joystick (Autodesk Fusion 360 design; units mm, degrees)
Autodesk Fusion 360 part; units mm, degrees
sketch "Sketch1" plane through (0, 0, 0) normal (0, 1, 0) x (1, 0, 0)
  line L0 (0, 0) -> (-17.5, 0)
  line L1 (-17.5, 0) -> (-17.5, -17.5)
  line L2 (-17.5, -17.5) -> (0, -17.5)
  line L3 (0, -17.5) -> (0, 0)
  dimension "d1" = 17.5
  dimension "d2" = 17.5
  constraint horizontal L0
  constraint vertical L1
  constraint horizontal L2
  constraint vertical L3
  constraint coincident L0.start L3.end
  measures "d1" distance of L0.start L2.end
  measures "d2" distance of L1.end L2.end
extrude "Extrude1" add sketch "Sketch1" along normal blind 11
sketch "Sketch2" plane through (0, 11, 0) normal (0, 1, 0) x (-1, 0, 0)
  line L0 (0, 17.5) -> (0, 0)
  line L1 (0, 0) -> (17.5, 0)
  line L2 (17.5, 0) -> (17.5, 17.5)
  line L3 (17.5, 17.5) -> (0, 17.5)
  line L4 (7.85, 9.3) -> (9.65, 9.3)
  line L5 (9.65, 9.3) -> (9.65, 8.2)
  line L6 (9.65, 8.2) -> (7.85, 8.2)
  line L7 (7.85, 8.2) -> (7.85, 9.3)
  line L8 (8.75, 9.3) -> (8.75, 8.2)
  line L9 (9.65, 8.75) -> (7.85, 8.75)
  line L10 (0, 17.5) -> (17.5, 17.5)
  line L11 (0, 17.5) -> (0, 0)
  line L12 (8.75, 17.5) -> (8.75, 0)
  line L13 (0, 8.75) -> (17.5, 8.75)
  dimension "d5" = 1.8
  dimension "d6" = 1.1
  constraint horizontal L4
  constraint vertical L5
  constraint horizontal L6
  constraint vertical L7
  constraint midpoint L4 L8.start
  constraint midpoint L6 L8.end
  constraint midpoint L5 L9.start
  constraint midpoint L7 L9.end
  constraint coincident L0.start L3.end
  constraint coincident L2.end L3.start
  constraint coincident L0.end L1.start
  constraint midpoint L10 L12.start
  constraint midpoint L1 L12.end
  constraint midpoint L0 L13.start
  constraint midpoint L2 L13.end
  constraint collinear L9 L13
  constraint collinear L8 L12
  measures "d5" distance of L4.start L4.end
  measures "d6" distance of L4.end L5.end
extrude "Extrude2" add sketch "Sketch2" along normal blind 8 contours L6 L7 L8 L9 L12 L13 | L4 L7 L8 L9 L12 L13 | L4 L5 L8 L9 L12 L13 | L5 L6 L8 L9 L12 L13
sketch "Sketch3" plane through (0, 0, 0) normal (1, 0, 0) x (0, 1, 0)
  line L0 (0, 17.5) -> (0, 0)
  line L1 (0, 0) -> (11, 0)
  line L2 (11, 0) -> (11, 17.5)
  line L3 (11, 17.5) -> (0, 17.5)
  line L4 (0, 13.75) -> (11, 13.75)
  line L5 (11, 13.75) -> (11, 3.75)
  line L6 (11, 3.75) -> (0, 3.75)
  line L7 (0, 3.75) -> (0, 13.75)
  line L8 (11, 8.75) -> (0, 8.75)
  line L9 (11, 17.5) -> (11, 0)
  line L10 (11, 8.75) -> (0, 8.75)
  dimension "d11" = 10
  dimension "d12" = 11
  constraint horizontal L4
  constraint vertical L5
  constraint horizontal L6
  constraint vertical L7
  constraint coincident L0 L4.start
  constraint midpoint L5 L8.start
  constraint midpoint L7 L8.end
  constraint coincident L2.end L3.start
  constraint coincident L1.end L2.start
  constraint midpoint L9 L8.start
  constraint midpoint L0 L8.end
  constraint collinear L8 L10
  measures "d11" distance of L4 L6
  measures "d12" distance of L5.end L6.end
extrude "Extrude3" add sketch "Sketch3" along normal blind 3.5 contours L0 L2 L4 L5 L7 L8 L9 L10 | L0 L2 L5 L6 L7 L8 L9 L10
sketch "Sketch4" plane through (0, 0, 17.5) normal (0, 0, 1) x (-1, 0, 0)
  line L0 (17.5, 0) -> (0, 0)
  line L1 (0, 0) -> (0, -11)
  line L2 (0, -11) -> (17.5, -11)
  line L3 (17.5, -11) -> (17.5, 0)
  line L4 (14.25, -11) -> (3.25, -11)
  line L5 (3.25, -11) -> (3.25, 0)
  line L6 (3.25, 0) -> (14.25, 0)
  line L7 (14.25, 0) -> (14.25, -11)
  line L8 (8.75, -11) -> (8.75, 0)
  line L9 (17.5, -11) -> (0, -11)
  line L10 (8.75, -11) -> (8.75, 0)
  dimension "d18" = 11
  constraint horizontal L4
  constraint vertical L5
  constraint horizontal L6
  constraint vertical L7
  constraint coincident L0 L5.end
  constraint coincident L2 L4.start
  constraint midpoint L4 L8.start
  constraint midpoint L6 L8.end
  constraint coincident L2.end L3.start
  constraint coincident L1.end L2.start
  constraint midpoint L9 L8.start
  constraint midpoint L0 L8.end
  constraint collinear L8 L10
  measures "d18" distance of L4.start L4.end
extrude "Extrude4" add sketch "Sketch4" along normal blind 3.5 contours L0 L2 L4 L6 L7 L8 L9 L10 | L0 L2 L4 L5 L6 L8 L9 L10
sketch "Sketch5" plane through (0, 0, 0) normal (0, -1, 0) x (1, 0, 0)
  line L0 (0, 13.75) -> (0, 17.5)
  line L1 (0, 17.5) -> (-3.25, 17.5)
  line L2 (-3.25, 17.5) -> (-3.25, 21)
  line L3 (-3.25, 21) -> (-14.25, 21)
  line L4 (-14.25, 21) -> (-14.25, 17.5)
  line L5 (-14.25, 17.5) -> (-17.5, 17.5)
  line L6 (-17.5, 17.5) -> (-17.5, 0)
  line L7 (-17.5, 0) -> (0, 0)
  line L8 (0, 0) -> (0, 3.75)
  line L9 (0, 3.75) -> (3.5, 3.75)
  line L10 (3.5, 3.75) -> (3.5, 13.75)
  line L11 (3.5, 13.75) -> (0, 13.75)
  line L12 (-13.45, 20.7) -> (-4.05, 20.7)
  line L13 (-4.05, 20.7) -> (-4.05, 17.8)
  line L14 (-4.05, 17.8) -> (-13.45, 17.8)
  line L15 (-13.45, 17.8) -> (-13.45, 20.7)
  line L16 (0.3, 12.95) -> (3.2, 12.95)
  line L17 (3.2, 12.95) -> (3.2, 4.55)
  line L18 (3.2, 4.55) -> (0.3, 4.55)
  line L19 (0.3, 4.55) -> (0.3, 12.95)
  line L20 (0, 17.5) -> (0, 0)
  line L21 (-17.5, 17.5) -> (0, 17.5)
  dimension "d21" = 0.8
  dimension "d22" = 0.8
  dimension "d23" = 0.8
  dimension "d24" = 0.8
  dimension "d25" = 0.3
  dimension "d27" = 0.3
  dimension "d28" = 0.3
  dimension "d29" = 0.3
  constraint horizontal L12
  constraint vertical L13
  constraint horizontal L14
  constraint vertical L15
  constraint horizontal L16
  constraint vertical L17
  constraint horizontal L18
  constraint vertical L19
  measures "d21" distance of L4 L15
  measures "d22" distance of L2 L13
  measures "d23" distance of L11 L16
  measures "d24" distance of L9 L18
  measures "d25" distance of L10 L17
  measures "d27" distance of L19 L20
  measures "d28" distance of L3 L12
  measures "d29" distance of L14 L21
extrude "Extrude5" add sketch "Sketch5" along normal blind 3.5 contours L12 L13 L14 L15 | L16 L17 L18 L19
equation "d21 = d23"
equation "d22 = d23"
equation "d24 = d23"
equation "d27 = d25"
equation "d28 = d25"
equation "d29 = d25"
